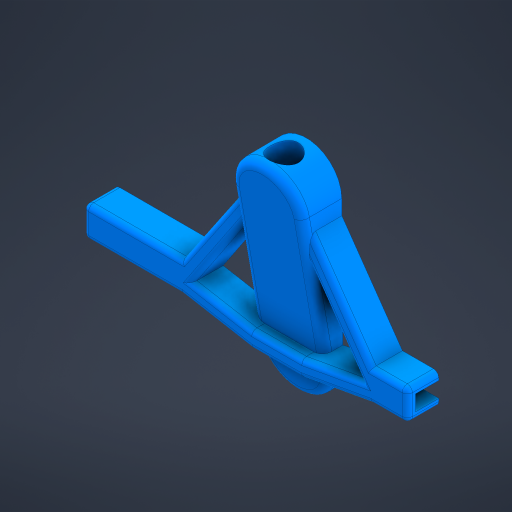
# Autodesk Inventor part: shaft_outlet
Saved by Autodesk Inventor 2024 (Build 280153000, 153)
## iProperties
Created: 2022-03-28
Part Number: shaft_outlet
Material: Generic
Document SubType Name: Modeling
Designer: kardo
Density: 1 g/cm^3
Appearance: Blue Plastic
Mass: 2.52542 g
Surface Area: 18.6998 cm^2
Volume: 2.52542 cm^3
Author: kardo
Autodesk Inventor part; units mm, degrees
ref_plane "YZ Plane" through (0, 0, 0) normal (1, 0, 0) x (0, 1, 0)
ref_plane "XZ Plane" through (0, 0, 0) normal (0, 1, 0) x (-1, 0, 0)
ref_plane "XY Plane" through (0, 0, 0) normal (0, 0, 1) x (1, 0, 0)
derived "stencil_frame.ipt"
sketch "sk_drivetrain_profile" plane through (6, 0, 0) normal (1, 0, 0) x (0, 1, 0)
  line L0 (-529.1844, 0) -> (410.1064, 0) construction
  line L1 (-345, 3089.1136) -> (-345, -1866.0023) construction
  line L2 (0, 3089.1136) -> (0, -1866.0023) construction
  line L3 (-140.3859, 53.0487) -> (-133.8494, 25.8223)
  line L4 (-377, 0) -> (-313.1973, 5.0214)
  line L5 (-137.1176, 39.4355) -> (-233.3061, 16.3427)
  line L6 (-296.4782, 6.3372) -> (-264.4984, 8.8541) construction
  line L7 (-264.4984, 8.8541) -> (-233.3061, 16.3427) construction
  line L8 (-133.8494, 25.8223) -> (-133.8494, 20.8223) construction
  line L9 (-313.1973, 5.0214) -> (-296.4782, 6.3372)
  line L10 (-850.7464, 3011.9134) -> (325.2296, -1886.3794) construction
  spline S0 degree 2 poles (-296.4782, 6.3372) (-264.4984, 8.8541) (-233.3061, 16.3427) knots 1 1 1 2 2 2
  line L11 (-233.9547, 19.044) -> (-137.7662, 42.1369) construction
  line L12 (-136.4691, 36.7341) -> (-232.6576, 13.6413) construction
  line L13 (-233.9547, 19.044) -> (-232.6576, 13.6413) construction
  line L14 (0, 21.3303) -> (-241.5001, 18.9703) construction
  line L15 (-55.7851, 21.5852) -> (-309.9218, 19.1017) construction
  point P0 (0, 0)
  point P1 (-221.5492, 19.1653)
  point P2 (-209.1437, 19.2865)
  point P3 (-205.6699, 20.1205)
sketch "sk_prop_shaft_cut" plane through (6, 0, 21.3303) normal (0, -0.0097716, 0.9999523) x (0, -0.9999523, -0.0097716)
  line L0 (233.9658, -4.7781) -> (205.6719, -4.7781)
  line L1 (233.9658, 4.7781) -> (205.6719, 4.7781)
  arc A0 (205.6719, 4.7781) -> (205.6719, -4.7781) centre (205.6719, 0) ccw
  arc A1 (233.9658, -4.7781) -> (233.9658, 4.7781) centre (233.9658, 0) ccw
  point P0 (0.2084, -6)
  point P1 (221.5598, 0)
  point P2 (209.1537, 0)
ref_plane "plane_motor_mount" through (0, -127.65, 0) normal (0, 0.9723699, 0.2334454) x (-1, 0, 0)
ref_plane "plane_prop_shaft_cut" through (6, 0, 21.3303) normal (0, -0.0097716, 0.9999523) x (0, -0.9999523, -0.0097716)
ref_plane "plane_tail_2" through (0, -230.0001, 0) normal (0, 1, 0) x (-1, 0, 0)
sketch "sk_long_inner" plane through (0, 0, 0) normal (1, 0, 0) x (0, 1, 0)
  line L0 (-483, 0) -> (357, 0) construction
  line L1 (-345, 107.6209) -> (-345, -224.5198) construction
  line L2 (-465, 54.4) -> (375, 54.4) construction
  line L3 (0, 107.6209) -> (0, -224.5198) construction
  line L4 (112.2, 107.6209) -> (112.2, -224.5198) construction
  line L5 (11.22, 28.832) -> (112.2, 28.832)
  line L6 (112.2, 37.536) -> (-345, 39.712)
  line L7 (11.22, 28.832) -> (-241.5001, 19.1524)
  line L8 (-241.5001, 19.1524) -> (-345, 16.32)
  line L9 (-345, 16.32) -> (112.2, 16.32) construction
  line L10 (112.2, 16.32) -> (112.2, 28.832) construction
  line L11 (-241.5001, 19.1524) -> (0, 21.3303)
  line L12 (0, 21.3303) -> (112.2, 28.832)
  line L13 (112.2, 37.536) -> (112.2, 28.832)
  line L14 (-114.9999, 107.6209) -> (-114.9999, -224.5198) construction
  line L15 (-230.0001, 107.6209) -> (-230.0001, -224.5198) construction
  line L16 (0, 21.3303) -> (0, 28.4023) construction
  point P0 (0, 0)
  point P1 (112.2, 22.576)
  point P2 (-345, 11.968)
derived "parameters_powertrain.ipt"
derived "parameters_frame.ipt"
derived "stencil_master.ipt"
ref_plane "plane_standoff_right" through (34.32, 0, 0) normal (1, 0, 0) x (0, 1, 0)
ref_plane "plane_standoff_left" through (-34.32, 0, 0) normal (1, 0, 0) x (0, 1, 0)
ref_plane "plane_upper_plate" through (6, -0.0078, 22.1302) normal (0, -0.0097716, 0.9999523) x (0, -0.9999523, -0.0097716)
extrude "lower_plate" add sketch "sk_prop_shaft_cut" along normal blind 0.8
sketch "sk_upper_plate" plane through (6, -233.9625, 19.844) normal (0, -0.0097716, 0.9999523) x (1, 0, 0)
  line L0 (-6.7781, 0) -> (-6.7781, 28.2939)
  arc A0 (6.7781, 28.2939) -> (-6.7781, 28.2939) centre (0, 28.2939) ccw
  line L1 (6.7781, 28.2939) -> (6.7781, 0)
  arc A1 (-6.7781, 0) -> (6.7781, 0) centre (0, 0) ccw
  line L2 (4.7781, 0) -> (4.7781, 28.2939) projected
  arc A2 (4.7781, 28.2939) -> (-4.7781, 28.2939) centre (0, 28.2939) ccw projected
  line L3 (-4.7781, 0) -> (-4.7781, 28.2939) projected
  arc A3 (-4.7781, 0) -> (4.7781, 0) centre (0, 0) ccw projected
  point P0 (-6, 233.7574)
  dimension "d29" = 2
  dimension "d30" = 2
  constraints: 4 end point, 4 point on circle, 2 centre point, 2 concentric, 2 tangent
  measures "d29" distance between parallel lines of L0 L3
  measures "d30" distance between parallel lines of L2 L1
extrude "upper_plate" add sketch "sk_upper_plate" along normal blind 8.89 contours L0 A0 L1 A1 | A3 L3 A2 L2
sketch "sk_trim" plane through (12.7781, -233.9625, 19.844) normal (1, 0, 0) x (0, 0.0097716, -0.9999523)
  line L0 (-1.9447, -6.7781) -> (-8.89, 35.0721)
  line L1 (0, 0) -> (0, -6.7781) projected
  line L2 (-8.89, 35.0721) -> (-8.89, 28.2939) projected
  line L3 (0, -6.7781) -> (-1.9447, -6.7781)
  line L4 (-1.9447, -6.7781) -> (-8.89, -6.7781)
  line L5 (-8.89, -6.7781) -> (-8.89, 28.2939)
  dimension "d16" = 1.9447
  constraints: 8 end point, 2 collinear, 1 perpendicular
  measures "d16" distance of L1.end L0.start
extrude "trim" cut sketch "sk_trim" against normal through all
fillet "main_fillet" radius 1.5 6 edges at (10.7929, -238.7773, 22.0712) (1.2071, -238.7773, 22.0712) (-0.7781, -219.8691, 25.3993) (1.2071, -200.9609, 28.7274) (10.7929, -200.9609, 28.7274) (12.7781, -219.8691, 25.3993)
sketch "sk_brace" plane through (6, -0.0078, 22.1302) normal (0, -0.0097716, 0.9999523) x (0, -0.9999523, -0.0097716)
  line L0 (230.0111, -49.848) -> (230.0111, 37.848) construction
  line L1 (-210.4436, -40.32) -> (475.1294, -40.32) construction
  line L2 (-210.4436, 28.32) -> (475.1294, 28.32) construction
  line L3 (211.348, -4.7781) -> (211.348, 4.7781)
  line L4 (205.6719, -4.7781) -> (205.6719, 4.7781)
  line L5 (233.9658, -4.7781) -> (233.9658, 4.7781)
  line L6 (230.7137, -4.7781) -> (230.7137, 4.7781)
  line L7 (233.9658, -4.7781) -> (205.6719, -4.7781) construction
  line L8 (233.9658, 4.7781) -> (205.6719, 4.7781) construction
  line L9 (231.5111, -18.32) -> (225.5111, -18.32) construction
  line L10 (225.5111, -18.32) -> (225.5111, -37.32)
  line L11 (231.5111, -37.32) -> (231.5111, -18.32)
  line L12 (233.9658, -4.7781) -> (231.5111, -18.32)
  line L13 (230.7137, -4.7781) -> (228.6119, -16.3729)
  line L14 (228.6119, -16.3729) -> (211.348, -4.7781)
  line L15 (225.5111, -18.32) -> (205.6719, -4.7781)
  line L16 (225.5111, -37.32) -> (231.5111, -37.32)
  line L17 (231.5111, 25.32) -> (231.5111, 18.32)
  line L18 (231.5111, 18.32) -> (233.9658, 4.7781)
  line L19 (205.6719, 4.7781) -> (225.5111, 18.32)
  line L20 (225.5111, 18.32) -> (225.5111, 25.32)
  line L21 (225.5111, 25.32) -> (231.5111, 25.32)
  line L22 (230.7137, 4.7781) -> (228.5814, 16.5413)
  line L23 (228.5814, 16.5413) -> (211.348, 4.7781)
  line L24 (231.5111, 18.32) -> (225.5111, 18.32) construction
  point P0 (0.2084, -6)
  point P1 (233.9658, 0)
  point P2 (205.6719, 0)
  point P3 (233.9658, 0)
  point P4 (205.6719, 0)
  dimension "d20" = 6
  dimension "d31" = 1.5
  dimension "d34" = 3
  dimension "d35" = 3
  dimension "d42" = 7
  dimension "d43" = 3.2
  dimension "d44" = 3.2
  constraints: 40 end point, 14 parallel, 5 point on line, 2 coincident, 2 collinear, 2 midpoint, 1 equal length, 1 perpendicular
  measures "d20" distance between parallel lines of L10 L11
  measures "d31" distance between parallel lines of L11 L0
  measures "d34" distance between parallel lines of L2 L21
  measures "d35" distance between parallel lines of L1 L16
  measures "d42" distance of L17.start L17.end
  measures "d43" distance between parallel lines of L19 L23
  measures "d44" distance between parallel lines of L18 L22
sketch3d "sk_sweep_axis"
  line L0 (-31.32, -231.5079, 19.868) -> (-31.32, -231.5079, 25.9352)
  dimension "d41" = 6.4
sweep "brace" add profiles "sk_brace" path "sk_sweep_axis" separate body
sketch "sk_carve_joint" plane through (-34.32, 0, 0) normal (1, 0, 0) x (0, 1, 0)
  line L0 (11.22, 28.832) -> (-241.5001, 19.1524) construction
  line L1 (-230.0001, 107.6209) -> (-230.0001, -224.5198) construction
  line L2 (-227.0001, 19.7078) -> (-227.0001, 24.3935)
  line L3 (-227.0001, 24.3935) -> (-230.0001, 24.3935)
  line L4 (-230.0001, 24.3935) -> (-230.0001, 19.5929)
  line L5 (-230.0001, 20.3935) -> (-229.9695, 19.5941) construction
  line L6 (-227.0001, 19.7078) -> (-230.0001, 19.5929)
  point P0 (0, 0)
  dimension "d36" = 3
  dimension "d37" = 0.8
  dimension "d38" = 4
  constraints: 10 end point, 4 point on line, 2 collinear, 2 perpendicular, 1 parallel
  measures "d36" distance of L2.end L3.end
  measures "d37" distance of L5.start L5.end
  measures "d38" distance from line of L5.start L3
extrude "carve_joint" add sketch "sk_carve_joint" along normal blind 7 separate body
mirror "mirror_carve_joint" about plane through (0, 0, 0) normal (1, 0, 0) bodies 3
combine bodies "sub_carve_joint" operation type subtract main body 2 bodies to subtract 3
fillet "brace_fillet" radius 1 22 edges at (-21.82, -231.5079, 25.9352) (17.5491, -232.7352, 25.9232) (27.82, -231.5079, 25.9352) (6, -233.9625, 25.9112) (-5.5491, -232.7352, 25.9232) (27.82, -225.5081, 25.9938) (17.5491, -215.589, 26.0907) (16.6597, -229.6444, 25.9534) (16.6597, -219.962, 26.048) (6, -230.7105, 25.9429) (-4.5755, -229.6596, 25.9532) (-4.5755, -219.9773, 26.0478) (-5.5491, -215.589, 26.0907) (-21.82, -225.5081, 25.9938) (6, -211.3457, 26.1322) (6, -205.6699, 26.1876) (31.32, -231.5079, 22.9016) (31.32, -225.5081, 22.9602) (31.32, -228.508, 25.9645) (-31.32, -231.5079, 22.9016) (-31.32, -225.5081, 22.9602) (-31.32, -228.508, 25.9645)
combine bodies "merge" operation type add bodies to combine 1 2
sketch "sk_drill" plane through (0, -127.65, 0) normal (0, 0.9723699, 0.2334454) x (-1, 0, 0)
  circle A0 centre (-6, 40.5561) radius 2.7781
  point P0 (0, -29.7993)
  dimension "d9" = 5.5563
  constraints: 1 centre point, 1 coincident
  measures "d9" diameter of A0
extrude "drill" cut sketch "sk_drill" along normal through all both and the other way through all bodies 1
equation "\"d4\" = shell_thickness"
equation "\"d7\" = 1.6 * prop_shaft_sleeve_od"
equation "\"d16\" = 0.35 * prop_shaft_sleeve_od"
equation "\"d31\" = -0.5 * bulkhead_thickness + 0.5 * d20"
equation "\"d34\" = bulkhead_thickness"
equation "\"d35\" = bulkhead_thickness"
equation "\"d36\" = bulkhead_thickness"
equation "\"d37\" = shell_thickness"
equation "\"d38\" = bulkhead_inset"
equation "\"d39\" = bulkhead_thickness + bulkhead_inset"
equation "\"d9\" = prop_shaft_sleeve_od"
equation "\"d28\" = shell_thickness"
equation "\"shell_thickness\" = 0.8"
equation "\"prop_shaft_sleeve_od\" = 5.55625"
equation "\"bulkhead_thickness\" = 3"
equation "\"bulkhead_inset\" = 4"
body "Solid1"
